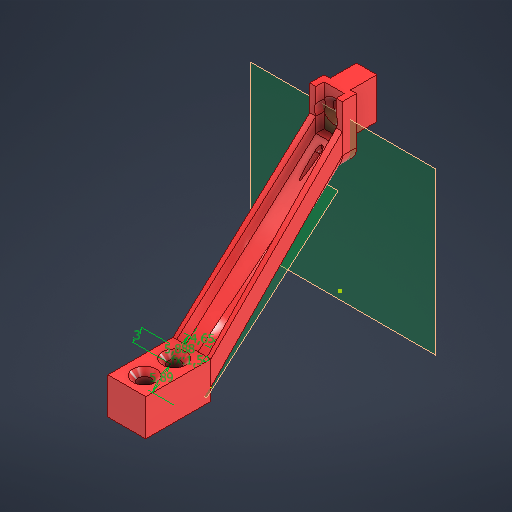
# Autodesk Inventor part: load_cell_bracket
Saved by Autodesk Inventor 2026 (Build 300175000, 175)
## iProperties
Created: 2025-04-29
Part Number: load_cell_bracket
Material: Generic
Document SubType Name: Modeling
Designer: Paul Juschitz
Density: 1 g/cm^3
Appearance: Light Red
Author: Paul Juschitz
Autodesk Inventor part; units mm, degrees
ref_plane "YZ Plane" through (0, 0, 0) normal (1, 0, 0) x (0, 1, 0)
ref_plane "XZ Plane" through (0, 0, 0) normal (0, 1, 0) x (-1, 0, 0)
ref_plane "XY Plane" through (0, 0, 0) normal (0, 0, 1) x (1, 0, 0)
sketch "Sketch1" plane through (0, 0, 0) normal (0, 1, 0) x (-1, 0, 0)
  line L0 (4.65, 8) -> (-4.65, 8)
  line L1 (-4.65, 8) -> (-4.65, -8)
  line L2 (-4.65, -8) -> (4.65, -8)
  line L3 (4.65, -8) -> (4.65, 8)
  line L4 (4.65, 8) -> (-4.65, -8) construction
  line L5 (-4.65, 8) -> (4.65, -8) construction
  point P0 (0, 0)
  dimension "d0" = 9.3
  dimension "d1" = 16
  constraints: 12 end point, 2 midpoint, 2 parallel, 1 horizontal, 1 perpendicular
  measures "d0" distance of L1.end L2.end
  measures "d1" distance of L0.end L1.end
extrude "Extrusion1" add sketch "Sketch1" along normal blind 6
sketch "Sketch2" plane through (0, 6, 0) normal (0, 1, 0) x (1, 0, 0)
  line L0 (-4.65, -8) -> (4.65, -8) projected
  line L1 (0, -8) -> (0, 8)
  line L2 (4.65, 8) -> (-4.65, 8) projected
  line L3 (-4.65, 8) -> (-4.65, -8) projected
  line L4 (-4.65, 0) -> (4.051, 0)
  point P0 (0, 0)
  point P1 (0, 3.65)
  point P2 (0, -3.65)
  dimension "d4" = 7.3
  constraints: 4 end point, 3 midpoint, 1 horizontal, 1 point on line, 1 symmetric about line
  measures "d4" distance of point (0, 3.65) point (0, -3.65)
hole "Hole1" at (0, 6, -3.65) at (0, 6, 3.65) direction (0, -1, 0) diameter 3.1 end through all countersink diameter 5.7 countersink angle 90
ref_plane "Work Plane1" through (4.65, 0, -43) normal (0, 0, -1) x (-1, 0, 0)
sketch "Sketch4" plane through (4.65, 0, -43) normal (0, 0, -1) x (-1, 0, 0)
  line L0 (0, 0) -> (0, 6) construction
  line L1 (0, 6) -> (9.3, 6) construction
  line L2 (0, 0) -> (9.3, 0) construction
  line L3 (4.65, 33.0442) -> (4.65, -21.0442) construction
  line L4 (2.15, 44) -> (7.15, 44)
  line L5 (7.15, 44) -> (7.15, 34)
  line L6 (7.15, 34) -> (2.15, 34)
  line L7 (2.15, 34) -> (2.15, 44)
  line L8 (2.15, 44) -> (7.15, 34) construction
  line L9 (7.15, 44) -> (2.15, 34) construction
  point P0 (4.65, 0)
  point P1 (4.65, 6)
  point P2 (4.65, 39)
  dimension "d21" = 10
  dimension "d22" = 5
  dimension "d28" = 28
  constraints: 14 end point, 4 midpoint, 2 parallel, 1 horizontal, 1 perpendicular, 1 point on line, 1 vertical
  measures "d21" distance of L4.end L5.end
  measures "d22" distance of L5.end L6.end
  measures "d28" distance between parallel lines of L1 L6
sketch "Sketch8" plane through (4.65, 0, -8) normal (0, 0, -1) x (-1, 0, 0)
  point P0 (4.65, 0)
extrude "Extrusion2" add sketch "Sketch4" along normal blind 8
sketch "Sketch9" plane through (4.65, 0, -43) normal (0, 0, 1) x (1, 0, 0)
  line L0 (-7.15, 44) -> (-2.15, 44) projected
  line L1 (-2.15, 34) -> (-7.15, 34) projected
  line L2 (-7.15, 44) -> (-2.15, 34) construction
  line L3 (-2.15, 44) -> (-7.15, 34) construction
  point P0 (-4.65, 0)
  point P1 (-4.65, 39)
  constraints: 4 end point, 2 midpoint
hole "Hole2" at (0, 39, -43) direction (0, 0, -1) diameter 3.1 end through all countersink diameter 5.7 countersink angle 90
sketch "Sketch11" plane through (4.65, 0, -43) normal (0, 0, 1) x (1, 0, 0)
  line L0 (-7.15, 34) -> (-7.15, 44) projected
  line L1 (-7.15, 44) -> (-8.65, 44)
  line L2 (-8.65, 44) -> (-8.65, 32.5)
  arc A0 (-2.15, 40.3684) -> (-7.15, 40.3684) centre (-4.65, 39) ccw projected
  line L3 (-7.15, 44) -> (-7.15, 40.3684)
  line L4 (-7.15, 34) -> (-7.15, 37.6316)
  line L5 (-7.15, 34) -> (-2.15, 34)
  line L6 (-7.15, 44) -> (-2.15, 44) projected
  line L7 (-2.15, 40.3684) -> (-2.15, 44)
  line L8 (-4.65, 53.4686) -> (-4.65, 24.5314)
  arc A1 (-8.65, 32.5) -> (-4.65, 28.5) centre (-4.65, 32.5) ccw
  line L9 (-2.15, 37.6316) -> (-2.15, 34) projected
  arc A2 (-7.15, 40.3684) -> (-7.15, 37.6316) centre (-4.65, 39) ccw
  line L10 (-2.15, 44) -> (-0.65, 44)
  line L11 (-0.65, 44) -> (-0.65, 32.5)
  arc A3 (-4.65, 28.5) -> (-0.65, 32.5) centre (-4.65, 32.5) ccw
  arc A4 (-2.15, 37.6316) -> (-2.15, 40.3684) centre (-4.65, 39) ccw
  line L12 (-2.15, 34) -> (-2.15, 37.6316)
  line L13 (-2.15, 40.3684) -> (-2.15, 44)
  point P0 (-4.65, 0)
  point P1 (-4.65, 34)
  dimension "d45" = 1.5
  dimension "d46" = 1.5
  constraints: 22 end point, 8 point on circle, 4 centre point, 3 point on line, 2 horizontal, 2 midpoint, 2 symmetric about line, 2 vertical, 1 coincident, 1 collinear, 1 line through centre, 1 perpendicular, 1 tangent, 2 other
  measures "d45" distance of L0.end L1.end
  measures "d46" distance from line of L5 L2.end
extrude "Extrusion4" add sketch "Sketch11" along normal blind 2 and the other way blind 1.5 contours L5 L8 A1 L2 L1 L0 A2 | L5 L9 A4 L7 L10 L11 A3 L8
sketch "Sketch14" plane through (4.65, 0, -41) normal (0, 0, 1) x (1, 0, 0)
  line L0 (-2.15, 37.6316) -> (-2.15, 34) projected
  line L1 (-2.15, 37.6316) -> (-2.15, 34)
  line L2 (-7.15, 34) -> (-7.15, 44) projected
  line L3 (-7.15, 37.6316) -> (-7.15, 34)
  line L4 (-2.15, 34) -> (-7.15, 34) projected
  line L5 (-7.15, 34) -> (-2.15, 34)
  line L6 (-2.15, 37.6316) -> (-0.65, 37.6316)
  line L7 (-0.65, 32.5) -> (-0.65, 44) projected
  line L8 (-0.65, 37.6316) -> (-0.65, 32.5)
  line L9 (-4.65, 42.3243) -> (-4.65, 25.6757)
  line L10 (-7.15, 37.6316) -> (-7.15, 34)
  line L11 (-7.15, 37.6316) -> (-8.65, 37.6316)
  line L12 (-8.65, 32.5) -> (-8.65, 37.6316)
  line L13 (-2.15, 34) -> (-7.15, 34)
  arc A0 (-8.65, 32.5) -> (-0.65, 32.5) centre (-4.65, 32.5) ccw
  point P0 (-4.65, 0)
  point P1 (-4.65, 34)
  point P2 (-8.65, 44)
  dimension "d53" = 8.3243
  constraints: 20 end point, 5 collinear, 3 symmetric about line, 2 midpoint, 2 point on circle, 2 point on line, 2 tangent, 1 centre point, 1 horizontal, 1 parallel, 1 vertical
  measures "d53" distance from line of L9.start L4
loft "Loft2" add profiles "Sketch14" section 2 edges at (0, 0, -8) (-4.65, 3, -8) (0, 6, -8) (4.65, 3, -8)
sketch "Sketch15" plane through (4.65, 0, -41) normal (0, 0, 1) x (1, 0, 0)
  arc A0 (-7.15, 37.6316) -> (-2.15, 37.6316) centre (-4.65, 39) ccw construction
  line L0 (-4.65, 53.4276) -> (-4.65, 24.5724) construction
  circle A1 centre (-4.65, 32.5) radius 0.75
  arc A2 (-8.65, 32.5) -> (-0.65, 32.5) centre (-4.65, 32.5) ccw construction
  point P0 (-4.65, 0)
  dimension "d58" = 1.5
  constraints: 2 end point, 1 centre point, 1 coincident, 1 midpoint, 1 point on line, 1 vertical
  measures "d58" diameter of A1
ref_plane "Work Plane2" through (4.65, 0, -8) normal (0, -0.756823, -0.6536199) x (-1, 0, 0)
sketch "Sketch16" plane through (4.65, 0, -8) normal (0, -0.756823, -0.6536199) x (-1, 0, 0)
  line L0 (4.65, 5.8877) -> (4.65, -5.8898)
  circle A0 centre (4.65, 3) radius 0.75
  line L1 (0, 0) -> (9.3, 0) projected
  point P0 (4.65, -6.0546)
  point P1 (4.65, 0)
  dimension "d59" = 1.5
  dimension "d60" = 3
  dimension "d61" = 4.65
  dimension "d62" = 5.8877
  dimension "d63" = 5.8898
  constraints: 2 end point, 1 centre point, 1 point on line, 1 vertical
  measures "d59" diameter of A0
  measures "d60" distance from line of L1 A0.centre
  measures "d61" distance from line of L1.end L0
  measures "d62" distance from line of L0.start L1
  measures "d63" distance from line of L0.end L1
sketch "Sketch17" plane through (4.65, 0, -44.5) normal (0, 0, -1) x (-1, 0, 0)
  circle A0 centre (4.65, 32.5) radius 0.75 projected
  circle A1 centre (4.65, 32.5) radius 0.75
  point P0 (4.65, 0)
  point P1 (5.4, 32.5)
  constraints: 1 centre point, 1 coincident, 1 horizontal alignment, 1 other
sketch "Sketch18" plane through (0, 0, 0) normal (1, 0, 0) x (0, 1, 0)
  arc A0 (4.6593, -10.9116) -> (0.9969, -10.8737) centre (2.8094, -12.6984) ccw
  line L0 (4.6593, -10.9116) -> (31.9385, -39.153)
  line L1 (32.5, -44.5) -> (32.5, -41) projected
  line L2 (32.5, -40.5425) -> (32.5, -41)
  arc A1 (32.5, -40.5425) -> (31.9385, -39.153) centre (30.5, -40.5425) ccw
  point P0 (0, 0)
  point P1 (1.9609, -10.2705)
  dimension "d70" = 2
  dimension "d71" = 2.572
  dimension "d72" = 135.993
  dimension "d73" = 0.8793
  constraints: 5 point on circle, 4 end point, 3 tangent, 2 centre point, 1 collinear
  measures "d70" radius of A1
  measures "d71" radius of A0
  measures "d72" angle of L0 L1
  measures "d73" distance from line of L1.end L0
sweep "Sweep2" cut profiles "Sketch15" path "Sketch18" path curves L1 L2 A1 L0 A0
sketch "Sketch19" plane through (0, 0, 0) normal (0, -1, 0) x (1, 0, 0)
  circle A0 centre (0, 3.65) radius 1.55 projected
  circle A1 centre (0, -3.65) radius 1.55 projected
  line L0 (4.65, 8) -> (4.65, -8) projected
  line L1 (-4.65, 8) -> (4.65, 8) projected
  line L2 (-4.65, -8) -> (-4.65, 8) projected
  line L3 (4.65, -8) -> (-4.65, -8) projected
  point P0 (0, 0)
extrude "Extrusion6" add sketch "Sketch19" along normal blind 3
equation "\"d58\" = wire_hole_diameter"
equation "\"d59\" = wire_hole_diameter"
equation "\"wire_hole_diameter\" = 1.5"
body "Solid1"
